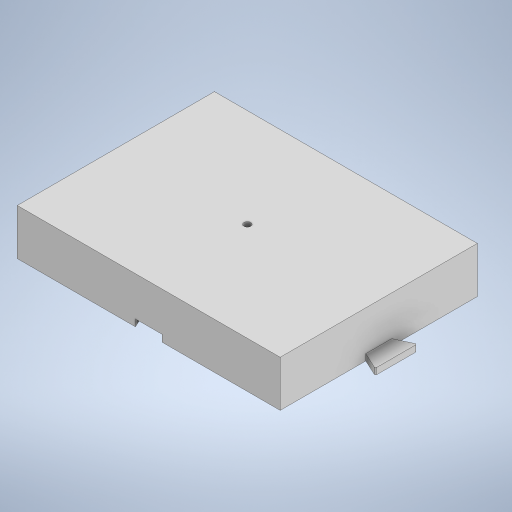
# Autodesk Inventor part: Area mh
Saved by Autodesk Inventor 2024 (Build 280153000, 153)
## iProperties
Created: 2024-03-01
Part Number: Area mh
Material: Generic
Document SubType Name: Modeling
Designer: laura
Density: 1 g/cm^3
Appearance: Default
Author: laura
Autodesk Inventor part; units mm, degrees
ref_plane "YZ Plane" through (0, 0, 0) normal (1, 0, 0) x (0, 1, 0)
ref_plane "XZ Plane" through (0, 0, 0) normal (0, 1, 0) x (-1, 0, 0)
ref_plane "XY Plane" through (0, 0, 0) normal (0, 0, 1) x (1, 0, 0)
sketch "Sketch1" plane through (0, 0, 0) normal (0, 1, 0) x (-1, 0, 0)
  line L0 (0, 0) -> (200, 0)
  line L1 (200, 0) -> (200, 150)
  line L2 (200, 150) -> (0, 150)
  line L3 (0, 150) -> (0, 0)
  line L4 (110.1274, 0) -> (89.8726, 0)
  line L5 (85.2304, 13.9946) -> (100, 13.9946)
  line L6 (89.8726, 0) -> (84.1428, 12.2875)
  arc A0 (85.2304, 13.9946) -> (84.1428, 12.2875) centre (85.2304, 12.7946) ccw
  line L7 (100, 13.9946) -> (114.7696, 13.9946)
  line L8 (110, 0.2) -> (110, 13.6303) construction
  arc A1 (115.8572, 12.2875) -> (114.7696, 13.9946) centre (114.7696, 12.7946) ccw
  line L9 (115.8572, 12.2875) -> (110.1274, 0)
  arc A2 (114.7696, 136.0054) -> (115.8572, 137.7125) centre (114.7696, 137.2054) ccw
  line L10 (100, 136.0054) -> (114.7696, 136.0054)
  line L11 (115.8572, 137.7125) -> (110.1274, 150)
  line L12 (110, 149.8) -> (110, 136.3697) construction
  line L13 (85.2304, 136.0054) -> (100, 136.0054)
  arc A3 (84.1428, 137.7125) -> (85.2304, 136.0054) centre (85.2304, 137.2054) ccw
  line L14 (110.1274, 150) -> (89.8726, 150)
  line L15 (89.8726, 150) -> (84.1428, 137.7125)
  line L16 (0.2, 85) -> (-13.2303, 85) construction
  line L17 (-13.1946, 75) -> (-13.1946, 89.7696)
  arc A4 (-12.0565, 90.4946) -> (-13.1946, 89.7696) centre (-12.3946, 89.7696) ccw
  line L18 (-12.0565, 90.4946) -> (0, 84.8726)
  line L19 (0, 84.8726) -> (0, 65.1274)
  line L20 (0, 65.1274) -> (-12.0565, 59.5054)
  arc A5 (-13.1946, 60.2304) -> (-12.0565, 59.5054) centre (-12.3946, 60.2304) ccw
  line L21 (-13.1946, 60.2304) -> (-13.1946, 75)
  point P0 (100, 0)
  point P1 (100, 150)
  point P2 (0, 75)
  point P3 (100, 0)
  point P4 (100, 0)
  point P5 (116.3393, 13.7946)
  point P6 (100, 0)
  point P7 (100, 150)
  point P8 (116.3393, 136.2054)
  point P9 (100, 150)
  point P10 (100, 150)
  point P11 (100, 150)
  point P12 (0, 75)
  point P13 (0, 75)
  point P14 (0, 75)
  point P15 (0, 75)
  dimension "d0" = 200
  dimension "d1" = 150
  dimension "d2" = 15
  constraints: 44 end point, 12 point on circle, 6 centre point, 5 midpoint, 2 parallel, 1 horizontal, 1 perpendicular
  measures "d0" distance of L2.end L1.end
  measures "d1" distance of L1.end L0.end
  measures "d2" distance of L8.start point (116.339, 13.795)
extrude "Extrusion1" add sketch "Sketch1" along normal blind 35 contours L3 L2 L15 A3 L13 L10 A2 L11 L1 L0 L9 A1 L7 L5 A0 L6 | L6 A0 L5 L7 A1 L9 L0 | L2 L11 A2 L10 L13 A3 L15
extrude "Extrusion2" cut sketch "Sketch1" along normal blind 5.2 contours L6 A0 L5 L7 A1 L9 L0 | L2 L11 A2 L10 L13 A3 L15
extrude "Extrusion3" add sketch "Sketch1" along normal blind 4.8 contours L20 A5 L21 L17 A4 L18 L3
sketch "Sketch2" plane through (0, 35, 0) normal (0, 1, 0) x (1, 0, 0)
  line L0 (0, -84.8726) -> (0, -65.1274) projected
  line L1 (-200, 0) -> (-200, -150) projected
  circle A0 centre (-100, -75) radius 2.6
  point P0 (0, 0)
  dimension "d9" = 5.2
  constraints: 1 centre point
  measures "d9" diameter of A0
extrude "Extrusion4" cut sketch "Sketch2" against normal blind 5.2
body "Solid1"
